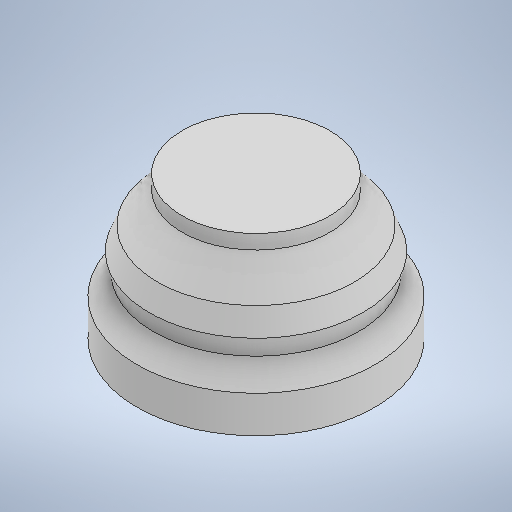
# Autodesk Inventor part: KINGHT BASE  medieum 1.0
Saved by Autodesk Inventor 2025.1 (Build 291241000, 241)
## iProperties
Created: 2024-10-24
Part Number: KINGHT BASE  medieum 1.0
Material: Genérico
Document SubType Name: Modeling
Designer: Octavio
Density: 1 g/cm^3
Appearance: Valor por defecto
Author: Octavio
Autodesk Inventor part; units mm, degrees
ref_plane "YZ Plane" through (0, 0, 0) normal (1, 0, 0) x (0, 1, 0)
ref_plane "XZ Plane" through (0, 0, 0) normal (0, 1, 0) x (-1, 0, 0)
ref_plane "XY Plane" through (0, 0, 0) normal (0, 0, 1) x (1, 0, 0)
sketch "Boceto2" plane through (0, 0, 0) normal (0, 0, 1) x (1, 0, 0)
  line L0 (-55.132, 97.6233) -> (57.4508, 97.6233) construction
  line L1 (57.4508, 97.6233) -> (57.4508, -13.0832) construction
  line L2 (57.4508, -13.0832) -> (-55.132, -13.0832) construction
  line L3 (-55.132, -13.0832) -> (-55.132, 97.6233) construction
  line L4 (0, 0) -> (0, 27.5828)
  line L5 (0, 27.5828) -> (0, 0)
  line L6 (-22.8755, 0.7881) -> (-22.8755, 7.0927)
  line L7 (-22.8755, 7.0927) -> (-19.7232, 11.0331)
  line L8 (-19.7232, 11.0331) -> (-20.5113, 14.5795)
  line L9 (-20.5113, 14.5795) -> (-18.9351, 18.9139)
  line L10 (-18.9351, 18.9139) -> (-17.0437, 21.2782)
  line L11 (-17.0437, 21.2782) -> (-15.7828, 22.8543)
  line L12 (-15.7828, 22.8543) -> (-14.2066, 24.8245)
  line L13 (-14.2066, 24.8245) -> (-14.2066, 27.5828)
  line L14 (-14.2066, 27.5828) -> (-12, 27.5828)
  line L15 (0, 27.5828) -> (-12, 27.5828)
  line L16 (-14.2066, 27.5828) -> (-12, 27.5828)
  line L17 (0, 0) -> (-22.8755, 0)
  line L18 (-22.8755, 0) -> (-22.8755, 0.7881)
  dimension "d18" = 12
  constraints: 30 end point, 3 point on line, 2 collinear, 2 horizontal, 2 parallel, 2 vertical, 1 perpendicular, 2 other
  measures "d18" distance of L14.end L4.end
revolve "Revolución1" add sketch "Boceto2" angle 360 about axis through (0, 0, 0) along (0, 1, 0)
